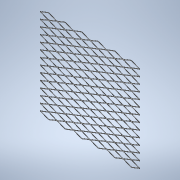
# Autodesk Inventor part: Expanded Metal STOCK
Saved by Autodesk Inventor 2020 (Build 240168000, 168)
## iProperties
Created: 2020-01-14
Part Number: Expanded Metal STOCK
Material: Generic
Document SubType Name: Modeling
Designer: aidan
Density: 1 g/cm^3
Appearance: Default
Author: aidan
Autodesk Inventor part; units mm, degrees
ref_plane "YZ Plane" through (0, 0, 0) normal (1, 0, 0) x (0, 1, 0)
ref_plane "XZ Plane" through (0, 0, 0) normal (0, 1, 0) x (-1, 0, 0)
ref_plane "XY Plane" through (0, 0, 0) normal (0, 0, 1) x (1, 0, 0)
sketch "Sketch1" plane through (0, 0, 0) normal (0, 0, 1) x (1, 0, 0)
  line L0 (-29.1905, 5.7934) -> (2.5595, 5.7934) construction
  line L1 (2.5595, 5.7934) -> (2.5595, -6.9066) construction
  line L2 (2.5595, -6.9066) -> (-29.1905, -6.9066) construction
  line L3 (-29.1905, -6.9066) -> (-29.1905, 5.7934) construction
  line L4 (-29.1905, -0.5566) -> (-27.9205, -0.5566) construction
  line L5 (-29.1905, 0.3959) -> (-27.9205, 0.3959)
  line L6 (-29.1905, -1.5091) -> (-27.9205, -1.5091)
  line L7 (-13.3155, 5.7934) -> (-13.3155, -6.9066) construction
  line L8 (2.5595, -0.5566) -> (1.2895, -0.5566) construction
  line L9 (2.5595, 0.3959) -> (1.2895, 0.3959)
  line L10 (2.5595, -1.5091) -> (1.2895, -1.5091)
  line L11 (-14.5855, 5.7934) -> (-12.0455, 5.7934)
  line L12 (-14.5855, -6.9066) -> (-12.0455, -6.9066)
  line L13 (-27.9205, 0.3959) -> (-14.5855, 5.7934)
  line L14 (-12.0455, 5.7934) -> (1.2895, 0.3959)
  line L15 (1.2895, -1.5091) -> (-12.0455, -6.9066)
  line L16 (-14.5855, -6.9066) -> (-27.9205, -1.5091)
  line L17 (-29.1905, 0.3959) -> (-29.1905, -1.5091)
  line L18 (2.5595, -1.5091) -> (2.5595, 0.3959)
  line L19 (0.9577, -0.5566) -> (-12.2417, -5.8992)
  line L20 (-12.2417, -5.8992) -> (-14.3894, -5.8992)
  line L21 (-14.3894, -5.8992) -> (-27.5888, -0.5566)
  line L22 (-27.5888, -0.5566) -> (-14.3894, 4.786)
  line L23 (-14.3894, 4.786) -> (-12.2417, 4.786)
  line L24 (-12.2417, 4.786) -> (0.9577, -0.5566)
  point P0 (0, 0)
  dimension "d0" = 12.7
  dimension "d1" = 31.75
  dimension "d2" = 15.875
  dimension "d3" = 1.905
  dimension "d4" = 2.54
  dimension "d5" = 1.27
  constraints: 50 end point, 8 symmetric about line, 6 parallel, 4 horizontal, 4 midpoint, 4 point on line, 1 collinear, 1 perpendicular, 6 other
  measures "d0" distance of L0.end L1.end
  measures "d1" distance of L0.start L0.end
  measures "d2" distance from line of L3 L7.start
  measures "d3" distance between parallel lines of L6 L5
  measures "d4" distance of L11.start L11.end
  measures "d5" distance of L5.start L5.end
extrude "Extrusion1" add sketch "Sketch1" along normal blind 0.254
pattern_linear "Rectangular Pattern1" count 14 spacing 12.7 along (0, 1, 0) count 6 spacing 31.75 along (1, 0, 0) of "Extrusion1"
body "Solid1"
